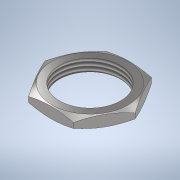
# Autodesk Inventor part: 16mm_nut
Saved by Autodesk Inventor 2020.2 (Build 242310000, 310)
## iProperties
Created: 2020-04-11
Part Number: 16mm_nut
Material: Stainless Steel
Document SubType Name: Modeling
Designer: agmlego
Mass: 3.02931 g
Surface Area: 5.64443 cm^2
Volume: 0.378664 cm^3
Density: 8 g/cm^3
Appearance: Semi-Polished
Author: agmlego
Autodesk Inventor part; units mm, degrees
ref_plane "YZ Plane" through (0, 0, 0) normal (1, 0, 0) x (0, 1, 0)
ref_plane "XZ Plane" through (0, 0, 0) normal (0, 1, 0) x (-1, 0, 0)
ref_plane "XY Plane" through (0, 0, 0) normal (0, 0, 1) x (1, 0, 0)
sketch "Sketch1" plane through (0, 0, 0) normal (0, 1, 0) x (-1, 0, 0)
  line L0 (10.9697, 0) -> (5.4848, -9.5)
  line L1 (5.4848, -9.5) -> (-5.4848, -9.5)
  line L2 (-5.4848, -9.5) -> (-10.9697, 0)
  line L3 (-10.9697, 0) -> (-5.4848, 9.5)
  line L4 (-5.4848, 9.5) -> (5.4848, 9.5)
  line L5 (5.4848, 9.5) -> (10.9697, 0)
  point P0 (0, 0)
  point P1 (0, 0)
  dimension "d0" = 19
  constraints: 12 end point, 1 coincident, 1 horizontal, 13 other
  measures "d0" distance between parallel lines of L1 L4
extrude "Extrusion1" add sketch "Sketch1" along normal blind 2.9
sketch "Sketch2" plane through (0, 2.9, 0) normal (0, 1, 0) x (1, 0, 0)
  point P0 (0, 0)
  point P1 (0, 0)
  constraints: 1 coincident
hole "Hole1" at (0, 2.9, 0) direction (0, -1, 0) diameter 14.9175 end through all thread size "M16x1" class "6H" standard "ANSI Metric M Profile"
sketch "Sketch4" plane through (0, 0, 0) normal (0, 0, 1) x (1, 0, 0)
  line L0 (5.4848, 2.9) -> (10.9697, 2.9) projected
  line L1 (10.9697, 2.9) -> (9.25, 2.9)
  line L2 (9.25, 2.9) -> (10.9697, 2.075)
  line L3 (10.9697, 0) -> (10.9697, 2.9) projected
  line L4 (10.9697, 2.075) -> (10.9697, 2.9)
  line L5 (10.9697, 0.825) -> (10.9697, 0)
  line L6 (10.9697, 0) -> (9.25, 0)
  line L7 (5.4848, 0) -> (10.9697, 0) projected
  line L8 (9.25, 0) -> (10.9697, 0.825)
  line L9 (-5.4848, 0) -> (5.4848, 0) construction
  line L10 (0, 0) -> (0, 5.9117) construction
  dimension "d10" = 1.25
  dimension "d11" = 9.25
  constraints: 14 end point, 5 point on line, 2 equal length, 2 perpendicular, 1 vertical
  measures "d10" distance of L5.start L2.end
  measures "d11" distance from line of L1.end L10
revolve "Revolution1" cut sketch "Sketch4" angle 360 about axis through (0, 0, 0) along (0, 1, 0)
body "Solid1"
